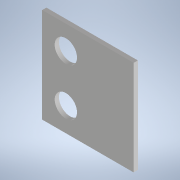
# Autodesk Inventor part: SP37V1 Suplemento Refuerzo
Saved by Autodesk Inventor 2021.2 (Build 252289000, 289)
## iProperties
Created: 2026-08-18
Part Number: SP37V1 Suplemento Refuerzo
Material: Generic
Document SubType Name: Modeling
Designer: nelso
Density: 1 g/cm^3
Appearance: Default
Author: nelso
Autodesk Inventor part; units mm, degrees
ref_plane "YZ Plane" through (0, 0, 0) normal (1, 0, 0) x (0, 1, 0)
ref_plane "XZ Plane" through (0, 0, 0) normal (0, 1, 0) x (-1, 0, 0)
ref_plane "XY Plane" through (0, 0, 0) normal (0, 0, 1) x (1, 0, 0)
sketch "Sketch1" plane through (0, 0, 0) normal (0, 1, 0) x (-1, 0, 0)
  line L0 (-13.5, 14) -> (13.5, 14)
  line L1 (13.5, 14) -> (13.5, -14)
  line L2 (13.5, -14) -> (-13.5, -14)
  line L3 (-13.5, -14) -> (-13.5, 14)
  line L4 (-13.5, 14) -> (13.5, -14) construction
  line L5 (13.5, 14) -> (-13.5, -14) construction
  point P0 (0, 0)
  dimension "d0" = 27
  dimension "d1" = 28
  constraints: 12 end point, 2 midpoint, 2 parallel, 1 horizontal, 1 perpendicular
  measures "d0" distance of L0.start L0.end
  measures "d1" distance of L0.end L1.end
extrude "Extrusion1" add sketch "Sketch1" along normal blind 1.25
sketch "Sketch2" plane through (0, 0, 0) normal (0, -1, 0) x (1, 0, 0)
  circle A0 centre (-6.5, 7) radius 3.3 projected
  circle A1 centre (-6.5, -7) radius 3.3 projected
  line L0 (-13.5, 14) -> (-13.5, -14) projected
  line L1 (19.5, -14) -> (-13.5, -14) projected
  line L2 (19.5, 14) -> (19.5, -14) projected
  line L3 (-13.5, 14) -> (19.5, 14) projected
  point P0 (0, 0)
hole "Hole1" at (-6.5, 0, 7) at (-6.5, 0, -7) direction (0, 1, 0) diameter 6.6 depth 8 tip angle 118 clearance for "Countersunk Flat Head Screw ISO 2009/7046" size "M6" standard "ISO"
body "Solid1"
